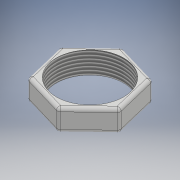
# Autodesk Inventor part: ANI
Saved by Autodesk Inventor 2017 (Build 210142000, 142)
## iProperties
Created: 2018-01-29
Part Number: ANI
Material: Generic
Document SubType Name: Modeling
Designer: CMRU-CAD-PC 8
Density: 1 g/cm^3
Appearance: Default
Author: CMRU-CAD-PC 8
Autodesk Inventor part; units mm, degrees
ref_plane "YZ Plane" through (0, 0, 0) normal (1, 0, 0) x (0, 1, 0)
ref_plane "XZ Plane" through (0, 0, 0) normal (0, 1, 0) x (-1, 0, 0)
ref_plane "XY Plane" through (0, 0, 0) normal (0, 0, 1) x (1, 0, 0)
sketch "Sketch1" plane through (0, 0, 0) normal (0, 0, 1) x (1, 0, 0)
  line L0 (-29.1128, -13.4147) -> (-38.6153, 25.6881)
  line L1 (-38.6153, 25.6881) -> (-9.5025, 53.4689)
  line L2 (-9.5025, 53.4689) -> (29.1128, 42.1469)
  line L3 (29.1128, 42.1469) -> (38.6153, 3.0441)
  line L4 (38.6153, 3.0441) -> (9.5025, -24.7367)
  line L5 (9.5025, -24.7367) -> (-29.1128, -13.4147)
  circle A0 centre (0, 14.3661) radius 30.9648
  point P0 (0, 0)
  constraints: 12 end point, 1 centre point, 1 coincident, 13 other
extrude "Extrusion1" add sketch "Sketch1" against normal blind 20
thread "Thread1" size "M50x3" class "6H" standard "ISO Metric profile" full length
fillet "Fillet1" radius 3 18 edges at (-29.1128, -13.4147, -10) (-38.6153, 25.6881, -10) (9.5025, -24.7367, -10) (38.6153, 3.0441, -10) (29.1128, 42.1469, -10) (-9.5025, 53.4689, -10) (-24.0589, 39.5785, -20) (9.8051, 47.8079, -20) (9.8051, 47.8079, 0) (-24.0589, 39.5785, 0) (33.864, 22.5955, 0) (33.864, 22.5955, -20) (-33.864, 6.1367, 0) (-33.864, 6.1367, -20) (-9.8051, -19.0757, -20) (-9.8051, -19.0757, 0) (24.0589, -10.8463, 0) (24.0589, -10.8463, -20)
body "Solid1"
